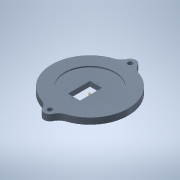
# Autodesk Inventor part: Onderste plaat bevestiging axiale lager
Saved by Autodesk Inventor 2021 (Build 250183000, 183)
## iProperties
Manager: Pierloot J.
Company: Emmaüs Bovenbouw Aalter
Created: 2015-08-18
Part Number: Onderste plaat bevestiging axiale lager
Material: S235
Catalog Web Link: http://emmausbovenbouw.op-weg.be/
Vendor: Emmaüsinstituut Bovenbouw Aalter
Document SubType Name: Modeling
Designer: Pierlootj
Engineer: Pierloot J.
Manufacturer: Standard
Standards Organization: Custom
Density: 7.86 g/cm^3
Appearance: Steel Blue
Title: Algemene titel
Subject: Specifieke titel
Author: Pierlootj
Keywords: Ruwe Ø xxxxx
Comments: Opmerking
Autodesk Inventor part; units mm, degrees
ref_plane "YZ Plane" through (0, 0, 0) normal (1, 0, 0) x (0, 1, 0)
ref_plane "XZ Plane" through (0, 0, 0) normal (0, 1, 0) x (-1, 0, 0)
ref_plane "XY Plane" through (0, 0, 0) normal (0, 0, 1) x (1, 0, 0)
sketch "Sketch2" plane through (0, 0, 0) normal (0, 0, 1) x (1, 0, 0)
  line L0 (0, 0) -> (0, 6)
  line L1 (0, 6) -> (-6, 6)
  line L2 (-6, 6) -> (6, 6)
  line L3 (6, 6) -> (6, -16.5)
  line L4 (6, -16.5) -> (-6, -16.5)
  line L5 (-6, -16.5) -> (-6, 6)
  circle A0 centre (0, 0) radius 40
  line L6 (6.3, 6.3) -> (-6.3, 6.3)
  line L7 (-6.3, 6.3) -> (-6.3, -16.8)
  line L8 (-6.3, -16.8) -> (6.3, -16.8)
  line L9 (6.3, -16.8) -> (6.3, 6.3)
  dimension "d15" = 6
  dimension "d16" = 6
  dimension "d17" = 12
  dimension "d18" = 22.5
  dimension "d19" = 80
  dimension "d20" = 0.3
  constraints: 20 end point, 4 parallel, 3 perpendicular, 1 centre point, 1 coincident, 1 horizontal, 1 vertical, 3 other
  measures "d15" distance of L0.start L0.end
  measures "d16" distance of L0.end L1.end
  measures "d17" distance of L3.end L4.end
  measures "d18" distance of L2.end L3.end
  measures "d19" diameter of A0
  measures "d20" distance between parallel lines of L2 L6
extrude "Extrusion4" add sketch "Sketch2" along normal blind 6.5 contours A0
sketch "Sketch3" plane through (0, 0, 6.5) normal (0, 0, 1) x (1, 0, 0)
  line L0 (-6.3, 6.3) -> (6.3, 6.3) projected
  line L1 (0, 6.3) -> (0, 8.25)
  circle A0 centre (0, 8.25) radius 0.5
  line L2 (6.3, -16.8) -> (-6.3, -16.8) projected
  line L3 (0, -16.8) -> (0, -18.75)
  circle A1 centre (0, -18.75) radius 0.5
  point P0 (0, 0)
  dimension "d23" = 1.95
  dimension "d24" = 1
  dimension "d25" = 1.95
  dimension "d26" = 1
  constraints: 4 end point, 2 centre point, 2 coincident, 2 midpoint, 2 vertical
  measures "d23" distance of L1.start L1.end
  measures "d24" diameter of A0
  measures "d25" distance of L3.start L3.end
  measures "d26" diameter of A1
extrude "Extrusion5" cut sketch "Sketch3" against normal blind 5.5
sketch "Sketch5" plane through (0, 0, 6.5) normal (0, 0, 1) x (1, 0, 0)
  circle A0 centre (0, 0) radius 40 projected
sketch "Sketch6" plane through (0, 0, 6.5) normal (0, 0, 1) x (1, 0, 0)
  line L0 (0, 0) -> (0, -42)
  line L1 (0, -42) -> (0, 42)
  circle A0 centre (0, 42) radius 2.5
  circle A1 centre (0, 42) radius 6
  circle A2 centre (0, -42) radius 2.5
  circle A3 centre (0, -42) radius 6
  dimension "d46" = 42
  dimension "d47" = 84
  dimension "d48" = 5
  dimension "d49" = 12
  dimension "d50" = 5
  dimension "d51" = 12
  constraints: 4 centre point, 4 coincident, 4 end point, 1 point on line, 1 vertical
  measures "d46" distance of L0.start L0.end
  measures "d47" distance of L0.end L1.end
  measures "d48" diameter of A0
  measures "d49" diameter of A1
  measures "d50" diameter of A2
  measures "d51" diameter of A3
extrude "Extrusion9" add sketch "Sketch6" against normal blind 6.5 contours A0 | A1 | A2 | A3
extrude "Extrusion10" cut sketch "Sketch6" against normal blind 6.5 contours A0 | A2
fillet "Fillet2" radius 12 4 edges at (-5.5074, -39.619, 3.25) (5.5074, -39.619, 3.25) (-5.5074, 39.619, 3.25) (5.5074, 39.619, 3.25)
sketch "Sketch8" plane through (0, 0, 6.5) normal (0, 0, 1) x (1, 0, 0)
  circle A0 centre (0, 0) radius 26.3
  dimension "d58" = 52.6
  constraints: 1 centre point, 1 coincident
  measures "d58" diameter of A0
extrude "Extrusion11" cut sketch "Sketch8" against normal blind 1.3
body "Solid4"
